Autodesk Inventor part; units mm, degrees
(part 2 of 2)
sketch "Sketch8" plane through (0, 0, 15.748) normal (0, 0, 1) x (1, 0, 0)
  spline S0 degree 4 poles (-26.2639, 14.356) (-23.3906, 14.8149) (-14.9027, 16.789) (-5.1775, 24.2035) (8.399, 20.9689) (12.1626, 21.0227) (15.3623, 18.6573) knots 0 0 0 0 0 0.432201 0.610065 1 1 1 1 1 projected
  spline S1 degree 4 poles (15.3623, 18.6573) (14.0844, 19.1095) (6.0457, 20.2504) (1.0033, 21.6252) (-13.688, 16.6903) (-14.6354, 16.5131) (-24.8081, 13.4817) (-26.2639, 14.356) knots 0 0 0 0 0 0.34942 0.500031 0.649154 1 1 1 1 1 projected
  spline S2 degree 4 poles (-58.3596, 12.6825) (-57.2325, 13.7843) (-51.9107, 17.5748) (-41.5573, 16.8573) (-38.56, 15.7519) (-36.7348, 15.5391) (-35.2387, 16.9945) (-32.33, 17.386) (-31.3664, 15.6515) (-30.3695, 15.3825) (-30.6352, 13.9476) knots 0 0 0 0 0 0.357484 0.480034 0.576415 0.657357 0.736723 0.814996 1 1 1 1 1 projected
  spline S3 degree 4 poles (-30.6352, 13.9476) (-30.9382, 14.2243) (-32.1883, 16.178) (-34.3185, 16.1348) (-36.0839, 15.0225) (-37.1207, 14.3376) (-39.694, 14.8986) (-41.6476, 15.3507) (-45.7698, 15.473) (-50.3637, 15.66) (-54.9604, 14.1617) (-57.2368, 12.3666) (-58.3596, 12.6825) knots 0 0 0 0 0 0.170055 0.237891 0.305971 0.377561 0.459955 0.555332 0.659577 0.768342 1 1 1 1 1 projected
  point P0 (0, 0)
extrude "Extrusion7" add sketch "Sketch8" along normal blind 0.508
sketch "Sketch9" plane through (0, 0, 12.7) normal (0, 0, 1) x (1, 0, 0)
  arc A0 (19.6488, -13.3581) -> (19.2729, -10.6088) centre (19.4518, -11.9847) ccw projected
  arc A1 (19.6488, -13.3581) -> (19.2729, -10.6088) centre (19.4518, -11.9847) ccw projected
  arc A2 (19.2729, -12.2118) -> (19.2729, -11.797) centre (19.2444, -12.0044) ccw projected
  arc A3 (19.2729, -12.2118) -> (19.2729, -11.797) centre (19.2444, -12.0044) ccw projected
  arc A4 (19.6488, -13.3581) -> (19.2729, -10.6088) centre (19.4518, -11.9847) ccw projected
  arc A5 (19.6488, -13.3581) -> (19.2729, -10.6088) centre (19.4518, -11.9847) ccw projected
  arc A6 (19.2729, -12.2118) -> (19.2729, -11.797) centre (19.2444, -12.0044) ccw projected
  arc A7 (19.2729, -12.2118) -> (19.2729, -11.797) centre (19.2444, -12.0044) ccw projected
  line L0 (56.7534, -28.0318) -> (56.7534, -31.1132) projected
  line L1 (55.4313, -31.1132) -> (55.4313, -28.0318) projected
  line L2 (55.4313, -28.0318) -> (56.7534, -28.0318) projected
  spline S0 degree 3 poles (56.7534, -31.1132) (56.7847, -31.9085) (55.4171, -32.9141) (54.2843, -33.0923) knots 0 0 0 0 1 1 1 1 projected
  spline S1 degree 2 poles (53.8931, -32.19) (55.2787, -31.9913) (55.4313, -31.1132) knots 0 0 0 1 1 1 projected
  line L3 (47.9942, -32.19) -> (53.8931, -32.19) projected
  line L4 (45.8846, -28.0318) -> (45.8846, -31.2446) projected
  spline S2 degree 2 poles (45.8846, -31.2446) (46.106, -31.8542) (47.9942, -32.19) knots 0 0 0 1 1 1 projected
  line L5 (44.5357, -28.0318) -> (45.8846, -28.0318) projected
  line L6 (44.5357, -28.0318) -> (44.5357, -31.2446) projected
  spline S3 degree 3 poles (44.5357, -31.2446) (44.5599, -32.2303) (45.931, -32.9686) (47.4288, -33.0923) knots 0 0 0 0 1 1 1 1 projected
  line L7 (47.4288, -33.0923) -> (54.2843, -33.0923) projected
  line L8 (68.5445, -29.0947) -> (59.7876, -29.0947) projected
  line L9 (59.7876, -30.2624) -> (68.5445, -30.2624) projected
  line L10 (59.7876, -29.0947) -> (59.7876, -30.2624) projected
  line L11 (59.7876, -31.2876) -> (67.2059, -31.2876) projected
  arc A8 (68.5445, -30.2624) -> (68.5445, -29.0947) centre (68.5073, -29.6785) ccw projected
  line L12 (59.7876, -33.0923) -> (59.7876, -31.2876) projected
  arc A9 (68.7933, -31.2876) -> (68.7933, -28.0318) centre (68.3545, -29.6597) ccw projected
  line L13 (72.2831, -33.0923) -> (71.0468, -33.0923) projected
  line L14 (69.228, -33.0923) -> (70.8153, -33.0923) projected
  line L15 (70.8153, -33.0923) -> (68.7933, -31.2876) projected
  line L16 (67.2059, -31.2876) -> (69.228, -33.0923) projected
  line L17 (58.6314, -28.0318) -> (58.6314, -33.0923) projected
  line L18 (58.6314, -33.0923) -> (59.7876, -33.0923) projected
  line L19 (58.6314, -28.0318) -> (68.7933, -28.0318) projected
  line L20 (96.8774, -33.0869) -> (85.9445, -33.0869) projected
  line L21 (87.1046, -31.9938) -> (96.8774, -31.9938) projected
  line L22 (96.8774, -31.9938) -> (96.8774, -33.0869) projected
  line L23 (98.2674, -31.6303) -> (98.2674, -32.5404) projected
  line L24 (109.6722, -28.4037) -> (109.6722, -29.3372) projected
  spline S4 degree 4 poles (109.6722, -28.4037) (108.7733, -28.0929) (105.6478, -27.7752) (103.1637, -27.669) (99.2636, -27.9958) (98.2311, -28.988) (98.1711, -29.9388) (99.4289, -31.0631) (101.7371, -30.9908) (105.1225, -30.9191) (107.0954, -30.7922) (108.598, -31.0126) (108.829, -31.6343) (107.9042, -32.2349) (105.4491, -32.1575) (101.0474, -32.2825) (98.7105, -31.9386) (98.2674, -31.6303) knots 0 0 0 0 0 0.176908 0.243948 0.300203 0.348723 0.396841 0.456186 0.523231 0.589094 0.644157 0.685091 0.722698 0.771731 0.835847 1 1 1 1 1 projected
  spline S5 degree 4 poles (98.2674, -32.5404) (99.5553, -33.0936) (102.1491, -32.7939) (106.7339, -33.9297) (110.1842, -32.5353) (110.0663, -30.5611) (108.6148, -30.0593) (106.1535, -29.9773) (102.3534, -29.9259) (101.0004, -30.198) (99.2528, -29.843) (99.5332, -29.1911) (100.6421, -28.7892) (102.2414, -28.7031) (108.031, -28.4051) (107.7183, -29.2242) (109.6722, -29.3372) knots 0 0 0 0 0 0.193476 0.265024 0.326054 0.382919 0.447483 0.515446 0.581924 0.636535 0.67795 0.716326 0.766204 0.827883 1 1 1 1 1 projected
  line L25 (76.9033, -28.0318) -> (78.9424, -28.0318) projected
  line L26 (78.5369, -28.7586) -> (77.5313, -28.7586) projected
  line L27 (85.9445, -28.0712) -> (87.1046, -28.0712) projected
  line L28 (77.5313, -28.7586) -> (75.3036, -30.7212) projected
  line L29 (80.5512, -30.7212) -> (78.5369, -28.7586) projected
  line L30 (75.3036, -30.7212) -> (80.5512, -30.7212) projected
  line L31 (81.8499, -31.6303) -> (73.975, -31.6303) projected
  line L32 (71.0468, -33.0923) -> (76.9033, -28.0318) projected
  line L33 (73.975, -31.6303) -> (72.2831, -33.0923) projected
  line L34 (87.1046, -28.0712) -> (87.1046, -31.9938) projected
  line L35 (83.6812, -33.0923) -> (81.8499, -31.6303) projected
  line L36 (78.9424, -28.0318) -> (85.281, -33.0923) projected
  line L37 (85.281, -33.0923) -> (83.6812, -33.0923) projected
  line L38 (85.9445, -33.0869) -> (85.9445, -28.0712) projected
  line L39 (-6.1614, -33.1318) -> (-7.5308, -33.1318) projected
  arc A10 (19.6488, -13.3581) -> (19.2729, -10.6088) centre (19.4518, -11.9847) ccw projected
  arc A11 (19.2729, -12.2118) -> (19.2729, -11.797) centre (19.2444, -12.0044) ccw projected
  line L40 (-6.1614, -28.9632) -> (-6.1614, -33.1318) projected
  line L41 (-0.8389, -28.9632) -> (-6.1614, -28.9632) projected
  line L42 (-7.5308, -33.1318) -> (-7.5308, -28.9632) projected
  line L43 (-12.884, -28.0712) -> (-0.8389, -28.0712) projected
  line L44 (-7.5308, -28.9632) -> (-12.884, -28.9632) projected
  line L45 (-12.884, -28.9632) -> (-12.884, -28.0712) projected
  line L46 (42.8837, -28.0318) -> (42.8837, -33.0923) projected
  line L47 (35.2952, -32.19) -> (41.2291, -28.0318) projected
  line L48 (36.1117, -33.3551) -> (34.439, -33.3551) projected
  line L49 (-14.4445, -33.1318) -> (-14.4445, -28.0712) projected
  line L50 (-16.0059, -33.1318) -> (-14.4445, -33.1318) projected
  line L51 (-14.4445, -28.0712) -> (-15.7205, -28.0712) projected
  line L52 (29.0483, -29.1342) -> (29.0483, -33.0923) projected
  line L53 (29.6369, -28.0318) -> (35.2952, -32.19) projected
  line L54 (41.6408, -33.0923) -> (41.6408, -29.0947) projected
  line L55 (41.6408, -29.0947) -> (36.1117, -33.3551) projected
  line L56 (42.8837, -33.0923) -> (41.6408, -33.0923) projected
  line L57 (41.2291, -28.0318) -> (42.8837, -28.0318) projected
  line L58 (34.439, -33.3551) -> (29.0483, -29.1342) projected
  line L59 (27.1651, -33.1318) -> (25.5653, -33.1318) projected
  line L60 (27.6953, -33.0923) -> (27.6953, -28.0318) projected
  line L61 (14.1671, -33.1318) -> (12.9309, -33.1318) projected
  line L62 (29.0483, -33.0923) -> (27.6953, -33.0923) projected
  line L63 (25.5653, -33.1318) -> (23.734, -31.6698) projected
  line L64 (23.734, -31.6698) -> (15.8591, -31.6698) projected
  line L65 (15.8591, -31.6698) -> (14.1671, -33.1318) projected
  line L66 (27.6953, -28.0318) -> (29.6369, -28.0318) projected
  line L67 (20.8265, -28.0712) -> (27.1651, -33.1318) projected
  line L68 (17.1877, -30.7607) -> (22.4353, -30.7607) projected
  arc A12 (10.4286, -30.3018) -> (10.4286, -29.1342) centre (10.3913, -29.718) ccw projected
  arc A13 (10.6774, -31.3271) -> (10.6774, -28.0712) centre (10.2386, -29.6991) ccw projected
  line L69 (12.9309, -33.1318) -> (18.7874, -28.0712) projected
  line L70 (22.4353, -30.7607) -> (20.4209, -28.798) projected
  line L71 (19.4154, -28.798) -> (17.1877, -30.7607) projected
  line L72 (18.7874, -28.0712) -> (20.8265, -28.0712) projected
  line L73 (20.4209, -28.798) -> (19.4154, -28.798) projected
  line L74 (0.5155, -28.0712) -> (10.6774, -28.0712) projected
  line L75 (10.4286, -29.1342) -> (1.6717, -29.1342) projected
  line L76 (1.6717, -29.1342) -> (1.6717, -30.3018) projected
  line L77 (1.6717, -30.3018) -> (10.4286, -30.3018) projected
  line L78 (1.6717, -31.3271) -> (9.09, -31.3271) projected
  line L79 (0.5155, -28.0712) -> (0.5155, -33.1318) projected
  line L80 (0.5155, -33.1318) -> (1.6717, -33.1318) projected
  line L81 (9.09, -31.3271) -> (11.1121, -33.1318) projected
  line L82 (12.6994, -33.1318) -> (10.6774, -31.3271) projected
  line L83 (11.1121, -33.1318) -> (12.6994, -33.1318) projected
  line L84 (-0.8389, -28.0712) -> (-0.8389, -28.9632) projected
  line L85 (1.6717, -33.1318) -> (1.6717, -31.3271) projected
  line L86 (-15.7205, -28.0712) -> (-15.7205, -31.9239) projected
  line L87 (-29.8009, -33.1318) -> (-29.8009, -28.0712) projected
  line L88 (-28.5736, -33.1318) -> (-29.8009, -33.1318) projected
  line L89 (-15.7205, -31.9239) -> (-24.4669, -28.0712) projected
  line L90 (-25.4696, -28.9632) -> (-16.0059, -33.1318) projected
  line L91 (-25.4696, -33.1318) -> (-25.4696, -28.9632) projected
  line L92 (-26.5667, -33.1318) -> (-25.4696, -33.1318) projected
  line L93 (-26.5667, -28.0712) -> (-26.5667, -33.1318) projected
  line L94 (-28.5736, -28.0712) -> (-28.5736, -33.1318) projected
  line L95 (-24.4669, -28.0712) -> (-26.5667, -28.0712) projected
  line L96 (-29.8009, -28.0712) -> (-28.5736, -28.0712) projected
  point P0 (0, 0)
  point P1 (115.6142, -40.8907)
  point P2 (9.341, -12.3982)
  point P3 (110.5342, -35.8107)
  point P4 (16.2097, -12.0534)
  point P5 (8.4273, -8.3923)
  point P6 (56.5057, -31.7819)
  point P7 (55.571, -32.5979)
  point P8 (55.069, -31.7453)
  point P9 (46.244, -31.638)
  point P10 (45.7794, -32.6766)
  point P11 (44.831, -31.9881)
  point P12 (98.3472, -29.1344)
  point P13 (99.0265, -28.404)
  point P14 (99.0804, -30.579)
  point P15 (99.2313, -31.9238)
  point P16 (99.4969, -29.6382)
  point P17 (99.5784, -29.3372)
  point P18 (100.2473, -29.9975)
  point P19 (100.2473, -28.9632)
  point P20 (100.4757, -32.9519)
  point P21 (101.4416, -27.8443)
  point P22 (101.4092, -28.7586)
  point P23 (101.4092, -30.9921)
  point P24 (102.0909, -30.0325)
  point P25 (102.9402, -32.1898)
  point P26 (98.3364, -29.7794)
  point P27 (104.5035, -27.7903)
  point P28 (104.4075, -33.2428)
  point P29 (105.1743, -28.6465)
  point P30 (105.4954, -30.8844)
  point P31 (106.3164, -29.9975)
  point P32 (106.8547, -32.1898)
  point P33 (107.6841, -28.0319)
  point P34 (107.7596, -30.9276)
  point P35 (108.3741, -33.0869)
  point P36 (108.2741, -31.9238)
  point P37 (108.579, -31.2446)
  point P38 (108.6544, -31.5419)
  point P39 (108.9267, -30.2624)
  point P40 (109.8893, -31.9935)
  point P41 (109.824, -30.8844)
  point P42 (107.7596, -28.9632)
  point P43 (115.6142, -40.8907)
  point P44 (-6.16, -14.8406)
  point P45 (14.2841, -13.7934)
  point P46 (-7.53, -11.2991)
  point P47 (5.0636, -11.3252)
  point P48 (-6.5969, -9.7072)
  point P49 (14.2529, -9.4349)
  point P50 (-10.3187, -12.2468)
  point P51 (-9.9687, -13.3581)
  point P52 (1.436, -12.3955)
  point P53 (0.5155, -13.3581)
  point P54 (-8.2602, -8.3913)
  point P55 (115.6142, -40.8907)
extrude "Extrusion8" add sketch "Sketch9" along normal blind 0.508
sketch "Sketch10" plane through (0, 0, 12.7) normal (0, 0, 1) x (1, 0, 0)
  line L0 (44.5357, -31.2446) -> (44.5357, -28.0318) projected
  line L1 (44.5357, -28.0318) -> (45.8846, -28.0318) projected
  line L2 (45.8846, -28.0318) -> (45.8846, -31.2446) projected
  line L3 (47.9942, -32.19) -> (53.8931, -32.19) projected
  line L4 (55.4313, -31.1132) -> (55.4313, -28.0318) projected
  line L5 (55.4313, -28.0318) -> (56.7534, -28.0318) projected
  line L6 (56.7534, -28.0318) -> (56.7534, -31.1132) projected
  line L7 (54.2843, -33.0923) -> (47.4288, -33.0923) projected
  line L8 (109.6722, -28.4037) -> (109.6722, -29.3372) projected
  line L9 (98.2674, -32.5404) -> (98.2674, -31.6303) projected
  line L10 (-28.5736, -33.1318) -> (-29.8009, -33.1318) projected
  line L11 (-29.8009, -33.1318) -> (-29.8009, -28.0712) projected
  line L12 (-29.8009, -28.0712) -> (-28.5736, -28.0712) projected
  line L13 (-28.5736, -28.0712) -> (-28.5736, -33.1318) projected
  line L14 (0.5155, -33.1318) -> (0.5155, -28.0712) projected
  line L15 (0.5155, -28.0712) -> (10.6774, -28.0712) projected
  arc A0 (10.6774, -31.3271) -> (10.6774, -28.0712) centre (10.2386, -29.6991) ccw projected
  line L16 (10.6774, -31.3271) -> (12.6994, -33.1318) projected
  line L17 (12.6994, -33.1318) -> (11.1121, -33.1318) projected
  line L18 (11.1121, -33.1318) -> (9.09, -31.3271) projected
  line L19 (9.09, -31.3271) -> (1.6717, -31.3271) projected
  line L20 (1.6717, -31.3271) -> (1.6717, -33.1318) projected
  line L21 (1.6717, -33.1318) -> (0.5155, -33.1318) projected
  line L22 (58.6314, -33.0923) -> (58.6314, -28.0318) projected
  line L23 (58.6314, -28.0318) -> (68.7933, -28.0318) projected
  arc A1 (68.7933, -31.2876) -> (68.7933, -28.0318) centre (68.3545, -29.6597) ccw projected
  line L24 (68.7933, -31.2876) -> (70.8153, -33.0923) projected
  line L25 (70.8153, -33.0923) -> (69.228, -33.0923) projected
  line L26 (69.228, -33.0923) -> (67.2059, -31.2876) projected
  line L27 (67.2059, -31.2876) -> (59.7876, -31.2876) projected
  line L28 (59.7876, -31.2876) -> (59.7876, -33.0923) projected
  line L29 (59.7876, -33.0923) -> (58.6314, -33.0923) projected
  line L30 (41.2291, -28.0318) -> (42.8837, -28.0318) projected
  line L31 (42.8837, -28.0318) -> (42.8837, -33.0923) projected
  line L32 (42.8837, -33.0923) -> (41.6408, -33.0923) projected
  line L33 (41.6408, -33.0923) -> (41.6408, -29.0947) projected
  line L34 (41.6408, -29.0947) -> (36.1117, -33.3551) projected
  line L35 (36.1117, -33.3551) -> (34.439, -33.3551) projected
  line L36 (34.439, -33.3551) -> (29.0483, -29.1342) projected
  line L37 (29.0483, -29.1342) -> (29.0483, -33.0923) projected
  line L38 (29.0483, -33.0923) -> (27.6953, -33.0923) projected
  line L39 (27.6953, -33.0923) -> (27.6953, -28.0318) projected
  line L40 (27.6953, -28.0318) -> (29.6369, -28.0318) projected
  line L41 (29.6369, -28.0318) -> (35.2952, -32.19) projected
  line L42 (35.2952, -32.19) -> (41.2291, -28.0318) projected
  line L43 (96.8774, -31.9938) -> (96.8774, -33.0869) projected
  line L44 (96.8774, -33.0869) -> (85.9445, -33.0869) projected
  line L45 (85.9445, -33.0869) -> (85.9445, -28.0712) projected
  line L46 (85.9445, -28.0712) -> (87.1046, -28.0712) projected
  line L47 (87.1046, -28.0712) -> (87.1046, -31.9938) projected
  line L48 (87.1046, -31.9938) -> (96.8774, -31.9938) projected
  line L49 (-14.4445, -28.0712) -> (-14.4445, -33.1318) projected
  line L50 (-14.4445, -33.1318) -> (-16.0059, -33.1318) projected
  line L51 (-16.0059, -33.1318) -> (-25.4696, -28.9632) projected
  line L52 (-25.4696, -28.9632) -> (-25.4696, -33.1318) projected
  line L53 (-25.4696, -33.1318) -> (-26.5667, -33.1318) projected
  line L54 (-26.5667, -33.1318) -> (-26.5667, -28.0712) projected
  line L55 (-26.5667, -28.0712) -> (-24.4669, -28.0712) projected
  line L56 (-24.4669, -28.0712) -> (-15.7205, -31.9239) projected
  line L57 (-15.7205, -31.9239) -> (-15.7205, -28.0712) projected
  line L58 (-15.7205, -28.0712) -> (-14.4445, -28.0712) projected
  line L59 (-6.1614, -28.9632) -> (-6.1614, -33.1318) projected
  line L60 (-6.1614, -33.1318) -> (-7.5308, -33.1318) projected
  line L61 (-7.5308, -33.1318) -> (-7.5308, -28.9632) projected
  line L62 (-7.5308, -28.9632) -> (-12.884, -28.9632) projected
  line L63 (-12.884, -28.9632) -> (-12.884, -28.0712) projected
  line L64 (-12.884, -28.0712) -> (-0.8389, -28.0712) projected
  line L65 (-0.8389, -28.0712) -> (-0.8389, -28.9632) projected
  line L66 (-0.8389, -28.9632) -> (-6.1614, -28.9632) projected
  line L67 (73.975, -31.6303) -> (72.2831, -33.0923) projected
  line L68 (72.2831, -33.0923) -> (71.0468, -33.0923) projected
  line L69 (71.0468, -33.0923) -> (76.9033, -28.0318) projected
  line L70 (76.9033, -28.0318) -> (78.9424, -28.0318) projected
  line L71 (78.9424, -28.0318) -> (85.281, -33.0923) projected
  line L72 (85.281, -33.0923) -> (83.6812, -33.0923) projected
  line L73 (83.6812, -33.0923) -> (81.8499, -31.6303) projected
  line L74 (81.8499, -31.6303) -> (73.975, -31.6303) projected
  line L75 (20.8265, -28.0712) -> (27.1651, -33.1318) projected
  line L76 (27.1651, -33.1318) -> (25.5653, -33.1318) projected
  line L77 (25.5653, -33.1318) -> (23.734, -31.6698) projected
  line L78 (23.734, -31.6698) -> (15.8591, -31.6698) projected
  line L79 (15.8591, -31.6698) -> (14.1671, -33.1318) projected
  line L80 (14.1671, -33.1318) -> (12.9309, -33.1318) projected
  line L81 (12.9309, -33.1318) -> (18.7874, -28.0712) projected
  line L82 (18.7874, -28.0712) -> (20.8265, -28.0712) projected
  arc A2 (-46.5779, -0.428) -> (-46.5779, -0.655) centre (-46.5512, -0.5415) ccw projected
  arc A3 (39.788, -6.6471) -> (39.6442, -4.2865) centre (39.6727, -5.4694) ccw projected
  arc A4 (-48.9231, -6.0144) -> (-49.0567, -6.4057) centre (-48.9661, -6.2182) ccw projected
  arc A5 (19.6488, -13.3581) -> (19.2729, -10.6088) centre (19.4518, -11.9847) ccw projected
  arc A6 (-53.5099, 18.2245) -> (-53.4631, 18.0644) centre (-53.4821, 18.1458) ccw projected
  line L83 (115.6142, -40.8907) -> (115.6142, 30.5334) projected
  line L84 (115.6142, 30.5334) -> (-107.6383, 30.5334) projected
  line L85 (-107.6383, 30.5334) -> (-107.6383, -40.8907) projected
  line L86 (-107.6383, -40.8907) -> (115.6142, -40.8907) projected
  line L87 (115.6142, -40.8907) -> (115.6142, 30.5334) projected
  line L88 (-107.6383, -40.8907) -> (115.6142, -40.8907) projected
  line L89 (-107.6383, 30.5334) -> (-107.6383, -40.8907) projected
  line L90 (115.6142, 30.5334) -> (-107.6383, 30.5334) projected
  line L91 (-107.6383, -40.8907) -> (115.6142, -40.8907) projected
  line L92 (-107.6383, -40.8907) -> (115.6142, -40.8907) projected
  line L93 (-107.6383, -40.8907) -> (115.6142, -40.8907) projected
  line L94 (-107.6383, -40.8907) -> (115.6142, -40.8907) projected
  line L95 (110.5342, -35.8107) -> (-102.5583, -35.8107) construction
  line L96 (110.5342, -35.8107) -> (-102.5583, -35.8107) construction
  line L97 (-107.6383, -40.8907) -> (115.6142, -40.8907) projected
  line L98 (-107.6383, -40.8907) -> (115.6142, 30.5334) construction
  line L99 (-102.5583, -35.8107) -> (-102.5583, 25.4534) construction
  line L100 (-102.5583, -35.8107) -> (-102.5583, 25.4534) construction
  line L101 (-59.868, -20.8988) -> (-55.6283, -20.8988) projected
  line L102 (-51.7454, -20.8988) -> (-51.7454, -24.6191) projected
  line L103 (-24.5946, -20.8988) -> (-51.7454, -20.8988) projected
  line L104 (-36.0253, -24.6191) -> (-24.5946, -24.6191) projected
  line L105 (-51.7454, -24.6191) -> (-40.4236, -24.6191) projected
  line L106 (-36.0253, -33.1318) -> (-36.0253, -24.6191) projected
  line L107 (-40.4236, -33.1318) -> (-36.0253, -33.1318) projected
  line L108 (-40.4236, -24.6191) -> (-40.4236, -33.1318) projected
  line L109 (-55.6283, -33.1318) -> (-59.868, -33.1318) projected
  line L110 (-59.868, -33.1318) -> (-59.868, -20.8988) projected
  line L111 (-55.6283, -20.8988) -> (-55.6283, -33.1318) projected
  line L112 (-101.4437, -24.341) -> (-96.395, -24.341) projected
  line L113 (-96.395, -24.341) -> (-96.395, -32.9519) projected
  line L114 (-96.395, -32.9519) -> (-92.1637, -32.9519) projected
  line L115 (-92.1637, -32.9519) -> (-92.1637, -25.7224) projected
  line L116 (-92.1637, -25.7224) -> (-80.2835, -34.0057) projected
  line L117 (-80.2835, -34.0057) -> (-68.147, -25.7224) projected
  line L118 (-68.147, -25.7224) -> (-68.147, -33.1318) projected
  line L119 (-68.147, -33.1318) -> (-63.961, -33.1318) projected
  line L120 (-63.961, -33.1318) -> (-63.961, -20.8988) projected
  line L121 (-63.961, -20.8988) -> (-68.4676, -20.8988) projected
  line L122 (-68.4676, -20.8988) -> (-80.2835, -28.9632) projected
  line L123 (-80.2835, -28.9632) -> (-91.8499, -20.8988) projected
  line L124 (-91.8499, -20.8988) -> (-101.4437, -20.8988) projected
  line L125 (-101.4437, -20.8988) -> (-101.4437, -24.341) projected
  line L126 (-107.6383, -40.8907) -> (115.6142, -40.8907) projected
  line L127 (-24.5946, -24.6191) -> (-24.5946, -20.8988) projected
  point P0 (0, 0)
  constraints: 20 other
extrude "Extrusion9" add sketch "Sketch10" along normal blind 1.016 contours L101 L111 L109 L110 | L103 L127 L104 L106 L107 L108 L105 L102 | L125 L124 L123 L122 L121 L120 L119 L118 L117 L116 L115 L114 L113 L112
sketch "Sketch11" plane through (0, 0, 12.7) normal (0, 0, 1) x (1, 0, 0)
  line L0 (-96.395, -24.341) -> (-96.395, -32.9519) projected
  line L1 (-96.395, -32.9519) -> (-92.1637, -32.9519) projected
  line L2 (-92.1637, -32.9519) -> (-92.1637, -25.7224) projected
  line L3 (-92.1637, -25.7224) -> (-80.2835, -34.0057) projected
  line L4 (-80.2835, -34.0057) -> (-68.147, -25.7224) projected
  line L5 (-68.147, -25.7224) -> (-68.147, -33.1318) projected
  line L6 (-68.147, -33.1318) -> (-63.961, -33.1318) projected
  line L7 (-63.961, -33.1318) -> (-63.961, -20.8988) projected
  line L8 (-63.961, -20.8988) -> (-68.4676, -20.8988) projected
  line L9 (-68.4676, -20.8988) -> (-80.2835, -28.9632) projected
  line L10 (-80.2835, -28.9632) -> (-91.8499, -20.8988) projected
  line L11 (-91.8499, -20.8988) -> (-101.4437, -20.8988) projected
  line L12 (-101.4437, -20.8988) -> (-101.4437, -24.341) projected
  line L13 (-101.4437, -24.341) -> (-96.395, -24.341) projected
  line L14 (-59.868, -33.1318) -> (-55.6283, -33.1318) projected
  line L15 (-55.6283, -33.1318) -> (-55.6283, -20.8988) projected
  line L16 (-55.6283, -20.8988) -> (-59.868, -20.8988) projected
  line L17 (-59.868, -20.8988) -> (-59.868, -33.1318) projected
  line L18 (-51.7454, -24.6191) -> (-40.4236, -24.6191) projected
  line L19 (-40.4236, -24.6191) -> (-40.4236, -33.1318) projected
  line L20 (-40.4236, -33.1318) -> (-36.0253, -33.1318) projected
  line L21 (-36.0253, -33.1318) -> (-36.0253, -24.6191) projected
  line L22 (-36.0253, -24.6191) -> (-24.5946, -24.6191) projected
  line L23 (-24.5946, -24.6191) -> (-24.5946, -20.8988) projected
  line L24 (-24.5946, -20.8988) -> (-51.7454, -20.8988) projected
  line L25 (-51.7454, -20.8988) -> (-51.7454, -24.6191) projected
  line L26 (-52.7614, -19.8828) -> (-23.5786, -19.8828)
  line L27 (-23.5786, -19.8828) -> (-23.5786, -25.6351)
  line L28 (-23.5786, -25.6351) -> (-35.0093, -25.6351)
  line L29 (-35.0093, -25.6351) -> (-35.0093, -34.1478)
  line L30 (-35.0093, -34.1478) -> (-41.4396, -34.1478)
  line L31 (-41.4396, -34.1478) -> (-41.4396, -25.6351)
  line L32 (-41.4396, -25.6351) -> (-52.7614, -25.6351)
  line L33 (-52.7614, -25.6351) -> (-52.7614, -19.8828)
  line L34 (-60.884, -19.8828) -> (-54.6123, -19.8828)
  line L35 (-54.6123, -19.8828) -> (-54.6123, -34.1478)
  line L36 (-54.6123, -34.1478) -> (-60.884, -34.1478)
  line L37 (-60.884, -34.1478) -> (-60.884, -19.8828)
  line L38 (-68.7813, -19.8828) -> (-62.945, -19.8828)
  line L39 (-62.945, -19.8828) -> (-62.945, -34.1478)
  line L40 (-62.945, -34.1478) -> (-69.163, -34.1478)
  line L41 (-69.163, -34.1478) -> (-69.163, -27.6459)
  line L42 (-69.163, -27.6459) -> (-80.2896, -35.2399)
  line L43 (-80.2896, -35.2399) -> (-91.1477, -27.6693)
  line L44 (-91.1477, -27.6693) -> (-91.1477, -33.9679)
  line L45 (-91.1477, -33.9679) -> (-97.411, -33.9679)
  line L46 (-97.411, -33.9679) -> (-97.411, -25.357)
  line L47 (-97.411, -25.357) -> (-102.4597, -25.357)
  line L48 (-102.4597, -25.357) -> (-102.4597, -19.8828)
  line L49 (-102.4597, -19.8828) -> (-91.5306, -19.8828)
  line L50 (-91.5306, -19.8828) -> (-80.2773, -27.7289)
  line L51 (-80.2773, -27.7289) -> (-68.7813, -19.8828)
  point P0 (0, 0)
  dimension "d70" = 1.016
  dimension "d71" = 1.016
  dimension "d72" = 1.016
  constraints: 52 end point, 23 other
  measures "d70" distance between parallel lines of L48 L12
  measures "d71" distance between parallel lines of L16 L34
  measures "d72" distance between parallel lines of L33 L25
extrude "Extrusion10" add sketch "Sketch11" along normal blind 0.508
fillet "Fillet1" radius 12.7 4 edges at (-107.6383, 30.5334, 6.35) (-107.6383, -40.8907, 6.35) (115.6142, 30.5334, 6.35) (115.6142, -40.8907, 6.35)
body "Solid1"
